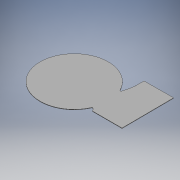
# Autodesk Inventor part: Solarpanel
Saved by Autodesk Inventor 2018 (Build 220112000, 112)
## iProperties
Created: 2018-04-27
Part Number: Solarpanel
Material: Siliziumnitrid
Document SubType Name: Modeling
Designer: gchri
Density: 3.18 g/cm^3
Appearance: Chrom - poliert - schwarz
Author: gchri
Autodesk Inventor part; units mm, degrees
ref_plane "YZ Plane" through (0, 0, 0) normal (1, 0, 0) x (0, 1, 0)
ref_plane "XZ Plane" through (0, 0, 0) normal (0, 1, 0) x (-1, 0, 0)
ref_plane "Arbeitsebene7" through (18.7798, 2.6465, 55.3142) normal (0, 0, 1) x (1, 0, 0)
sketch "Skizze6" plane through (18.7798, 2.6465, 55.3142) normal (0, 0, 1) x (1, 0, 0)
  arc A0 (-23.0224, 40.731) -> (-21.4881, -30.0932) centre (-96.7471, 3.7051) ccw
  line L0 (-13.4513, 86.676) -> (-13.5716, 68.19)
  line L1 (57.7529, -35.9083) -> (-12.3154, -35.9083)
  arc A1 (-19.3389, 40.9927) -> (-13.5716, 68.19) centre (-134.5985, 79.6442) ccw
  arc A2 (-14.2907, -34.2219) -> (-19.2239, -28.9615) centre (-20.6365, -35.2296) ccw
  arc A3 (-23.0224, 40.731) -> (-19.3389, 40.9927) centre (-21.2351, 41.6286) ccw
  arc A4 (-19.2239, -28.9615) -> (-21.4881, -30.0932) centre (-19.6636, -30.9126) ccw
  arc A5 (-14.2907, -34.2219) -> (-12.3154, -35.9083) centre (-12.3154, -33.9083) ccw
  line L2 (-180.3673, 88.095) -> (295.6199, 91.5808)
  line L3 (-13.4513, 86.676) -> (-13.4707, 89.3173)
  line L4 (-13.4707, 89.3173) -> (57.6263, 89.8379)
  line L5 (58.5471, -35.9083) -> (57.7529, -35.9083)
  line L6 (56.6011, 229.8342) -> (57.6263, 89.8379)
  line L7 (-13.4707, 89.3173) -> (57.6263, 89.8379)
  line L8 (57.6263, 89.8379) -> (58.5471, -35.9083)
  point P0 (-18.7798, -2.6465)
  point P1 (-97.992, 173.7006)
  dimension "d22" = 165
  dimension "d24" = 2
  dimension "d25" = 2
  constraints: 18 end point, 12 point on circle, 6 centre point, 6 tangent, 2 perpendicular, 1 coincident, 1 collinear, 1 equal radius, 1 midpoint, 1 point on line, 7 other
  measures "d22" diameter of A0
  measures "d24" radius of A3
  measures "d25" radius of A4
extrude "Extrusion6" add sketch "Skizze6" along normal blind 1
